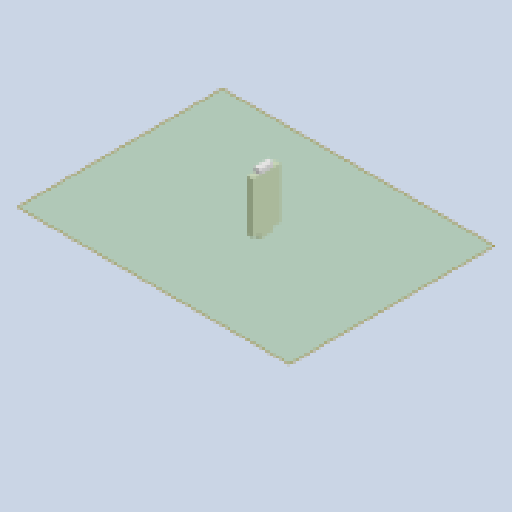
# Autodesk Inventor part: стенка 2
Saved by Autodesk Inventor 2024.2 (Build 282272000, 272)
## iProperties
Created: 2025-12-09
Part Number: стенка 2
Material: Типовые
Document SubType Name: Modeling
Designer: katya_notebook
Density: 1 g/cm^3
Appearance: По умолчанию
Author: katya_notebook
Autodesk Inventor part; units mm, degrees
ref_plane "YZ Plane" through (0, 0, 0) normal (1, 0, 0) x (0, 1, 0)
ref_plane "XZ Plane" through (0, 0, 0) normal (0, 1, 0) x (-1, 0, 0)
ref_plane "XY Plane" through (0, 0, 0) normal (0, 0, 1) x (1, 0, 0)
ref_plane "РабПлоскость1" through (-329.2239, 210.3045, -11.0538) normal (0, -1, 0) x (1, 0, 0)
sketch "Эскиз1" plane through (-329.2239, 210.3045, -11.0538) normal (0, -1, 0) x (1, 0, 0)
  line L0 (-46.5606, -73) -> (-52.5606, -73)
  line L1 (-52.5606, -73) -> (-52.5606, -43)
  line L2 (-52.5606, -43) -> (-46.5606, -43)
  line L3 (-46.5606, -43) -> (-46.5606, -73)
  line L4 (-23.55, -78) -> (-51.55, -78) projected
  point P0 (329.2239, 11.0538)
  dimension "d0" = 6
  dimension "d1" = 30
  dimension "d2" = 5
  constraints: 8 end point, 2 parallel, 1 horizontal, 1 perpendicular
  measures "d0" distance of L1.end L2.end
  measures "d1" distance of L0.end L1.end
  measures "d2" distance from line of L4 L0.start
ref_plane "РабПлоскость2" through (-464.2239, 154.5996, -124.0538) normal (0, 1, 0) x (0, 0, 1)
extrude "Выдавливание1" add sketch "Эскиз1" along normal up to surface (55.705 mm away)
sketch "Эскиз2" plane through (-375.7846, 210.3045, -54.0538) normal (1, 0, 0) x (0, 0, -1)
  line L0 (0, -55.705) -> (30, -55.705) projected
  line L1 (30, -55.705) -> (20.1565, -55.705)
  line L2 (20.1565, -55.705) -> (20.1565, -61.3199)
  line L3 (20.1565, -61.3199) -> (30, -61.3199)
  line L4 (30, -61.3199) -> (30, -55.705)
  line L5 (0, -55.705) -> (8.9015, -55.705)
  line L6 (8.9015, -55.705) -> (8.9015, -61.3199)
  line L7 (8.9015, -61.3199) -> (0, -61.3199)
  line L8 (0, -61.3199) -> (0, -55.705)
  line L9 (18.4286, -53.3384) -> (11.9286, -53.3384)
  line L10 (11.9286, -53.3384) -> (11.9286, -50.3384)
  line L11 (11.9286, -50.3384) -> (18.4286, -50.3384)
  line L12 (18.4286, -50.3384) -> (18.4286, -53.3384)
  point P0 (-54.0538, -210.3045)
  point P1 (22.5, -55.705)
  dimension "d13" = 6.5
  dimension "d14" = 3
  constraints: 24 end point, 6 parallel, 3 horizontal, 3 perpendicular, 2 point on line
  measures "d13" distance of L9.start L9.end
  measures "d14" distance of L11.end L9.start
extrude "Выдавливание2" [suppressed]
sketch "Эскиз3" plane through (-375.7846, 154.5996, -84.0538) normal (1, 0, 0) x (0, 0, -1)
  point P0 (-84.0538, -154.5996)
